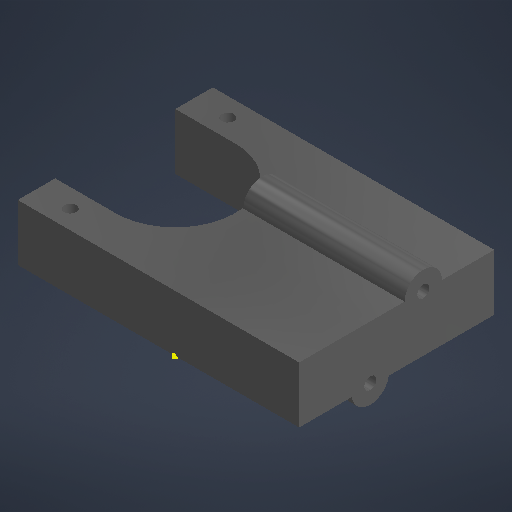
# Autodesk Inventor part: braket motor1
Saved by Autodesk Inventor 2026.2 (Build 302298010, 298A)
## iProperties
Part Number: braket motor1
Material: Generic
Document SubType Name: Modeling
Designer: acer
Appearance: Default
Author: acer
Autodesk Inventor part; units mm, degrees
ref_plane "YZ Plane" through (0, 0, 0) normal (1, 0, 0) x (0, 1, 0)
ref_plane "XZ Plane" through (0, 0, 0) normal (0, 1, 0) x (-1, 0, 0)
ref_plane "XY Plane" through (0, 0, 0) normal (0, 0, 1) x (1, 0, 0)
sketch "Sketch4" plane through (0, 0, 0) normal (0, 1, 0) x (-1, 0, 0)
  line L0 (0, 0) -> (-42, 0)
  line L1 (-42, 0) -> (-42, -52)
  line L2 (-42, -52) -> (0, -52)
  line L3 (0, -52) -> (0, 0)
  dimension "d79" = 42
  dimension "d80" = 52
  constraints: 8 end point, 2 parallel, 1 horizontal, 1 perpendicular
  measures "d79" distance of L2.end L1.end
  measures "d80" distance of L1.end L0.end
extrude "Extrusion4" add sketch "Sketch4" along normal blind 15
sketch "Sketch5" plane through (0, 15, 0) normal (0, 1, 0) x (1, 0, 0)
  line L0 (0, 0) -> (0, 10)
  line L1 (0, 52) -> (0, 0) projected
  line L2 (0, 52) -> (0, 42)
  circle A0 centre (16, 26) radius 16
  line L3 (42, 0) -> (42, 52) projected
  line L4 (0, 10) -> (42, 10)
  line L5 (0, 42) -> (42, 42)
  point P0 (42, 26)
  point P1 (16, 10)
  point P2 (16, 42)
  dimension "d83" = 10
  dimension "d84" = 10
  dimension "d93" = 32
  dimension "d94" = 26
  constraints: 8 end point, 4 point on line, 2 perpendicular, 1 centre point, 1 midpoint
  measures "d83" distance of L0.start L0.end
  measures "d84" distance of L1.start L2.end
  measures "d93" diameter of A0
  measures "d94" distance of point (42, 26) A0.centre
extrude "Extrusion5" cut sketch "Sketch5" against normal blind 15 contours L5 A0 L1 | A0 L4 L1 | A0
sketch "Sketch10" plane through (42, 0, 0) normal (1, 0, 0) x (0, 0, -1)
  circle A0 centre (5, 7.5) radius 2.65 projected
  line L0 (18.9423, 0.7517) -> (33.0845, 14.8938)
  line L1 (0, 0) -> (52, 0) projected
  line L2 (26, 0) -> (26, 15)
  line L3 (0, 15) -> (52, 15) projected
  line L4 (18.9423, 0.7517) -> (26.0134, 7.8228)
  circle A1 centre (18.9423, 0.7517) radius 1.55
  circle A2 centre (33.0845, 14.8938) radius 1.55
  circle A3 centre (33.0845, 14.8938) radius 5
  circle A4 centre (18.9423, 0.7517) radius 5
  line L5 (52, 0) -> (0, 0)
  point P0 (38.0833, 15)
  point P1 (28.0856, 15)
  point P2 (31.5381, 15)
  point P3 (34.6308, 15)
  point P4 (13.9992, 0)
  point P5 (23.8855, 0)
  point P6 (20.2979, 0)
  point P7 (17.5868, 0)
  point P8 (47, 7.5)
  dimension "d115" = 20
  dimension "d116" = 3.1
  dimension "d117" = 3.1
  dimension "d118" = 10
  dimension "d119" = 10
  constraints: 8 end point, 4 centre point, 4 coincident, 3 midpoint, 3 symmetric about line
  measures "d115" distance of L0.start L0.end
  measures "d116" diameter of A1
  measures "d117" diameter of A2
  measures "d118" diameter of A3
  measures "d119" diameter of A4
extrude "Extrusion10" add sketch "Sketch10" against normal blind 10 contours A1 L1 A4 | A3 L3 A2
sketch "Sketch11" plane through (42, 0, 0) normal (1, 0, 0) x (0, 0, -1)
  arc A0 (34.6308, 15) -> (31.5381, 15) centre (33.0845, 14.8938) ccw projected
  circle A1 centre (33.0845, 14.8938) radius 1.55
  point P0 (0, 0)
  point P1 (31.5381, 15)
  point P2 (34.6308, 15)
  dimension "d122" = 3.1
  constraints: 1 centre point, 1 coincident
  measures "d122" diameter of A1
extrude "Extrusion11" cut sketch "Sketch11" against normal blind 30
sketch "Sketch12" plane through (42, 0, 0) normal (1, 0, 0) x (0, 0, -1)
  circle A0 centre (33.0845, 14.8938) radius 1.55 projected
  circle A1 centre (33.0845, 14.8938) radius 3
  point P0 (0, 0)
  dimension "d125" = 6
  constraints: 1 centre point, 1 coincident
  measures "d125" diameter of A1
extrude "Extrusion12" cut sketch "Sketch12" against normal blind 30
sketch "Sketch13" plane through (42, 0, 0) normal (1, 0, 0) x (0, 0, -1)
  circle A0 centre (33.0845, 14.8938) radius 3 projected
  circle A1 centre (33.0845, 14.8938) radius 1.625
  point P0 (0, 0)
  dimension "d128" = 3.25
  constraints: 1 centre point, 1 coincident
  measures "d128" diameter of A1
extrude "Extrusion13" add sketch "Sketch13" against normal blind 5
sketch "Sketch14" plane through (42, 0, 0) normal (1, 0, 0) x (0, 0, -1)
  arc A0 (17.5868, 0) -> (20.2979, 0) centre (18.9423, 0.7517) ccw projected
  circle A1 centre (18.9423, 0.7517) radius 3
  point P0 (0, 0)
  dimension "d131" = 6
  constraints: 1 centre point, 1 coincident
  measures "d131" diameter of A1
extrude "Extrusion14" cut sketch "Sketch14" against normal blind 16
sketch "Sketch15" plane through (42, 0, 0) normal (1, 0, 0) x (0, 0, -1)
  circle A0 centre (18.9423, 0.7517) radius 1.625
  circle A1 centre (18.9423, 0.7517) radius 2.65
  point P0 (0, 0)
  dimension "d134" = 3.25
  constraints: 2 centre point, 2 coincident
  measures "d134" diameter of A0
extrude "Extrusion15" add sketch "Sketch15" against normal blind 5
sketch "Sketch16" plane through (42, 0, -52) normal (1, 0, 0) x (0, 0, -1)
  arc A0 (-20.2979, 0) -> (-17.5868, 0) centre (-18.9423, 0.7517) ccw projected
  circle A1 centre (-18.9423, 0.7517) radius 1.55
  point P0 (-52, 0)
  constraints: 1 centre point, 1 coincident
sketch "Sketch18" plane through (0, 0, 0) normal (0, -1, 0) x (1, 0, 0)
  line L0 (0, -10) -> (0, 0) projected
  line L1 (0, -5) -> (9, -5)
  circle A0 centre (9, -5) radius 1.625
  line L2 (0, -52) -> (0, -42) projected
  line L3 (0, -47) -> (9, -47)
  circle A1 centre (9, -47) radius 1.625
  dimension "d144" = 9
  dimension "d145" = 3.25
  dimension "d146" = 9
  dimension "d147" = 3.25
  constraints: 4 end point, 2 centre point, 2 coincident, 2 horizontal, 2 midpoint
  measures "d144" distance of L1.start L1.end
  measures "d145" diameter of A0
  measures "d146" distance of L3.start L3.end
  measures "d147" diameter of A1
extrude "Extrusion17" cut sketch "Sketch18" against normal blind 26.5
sketch "Sketch19" plane through (42, 0, 0) normal (1, 0, 0) x (0, 0, -1)
  point P0 (0, 0)
sketch "Sketch20" plane through (42, 0, 0) normal (1, 0, 0) x (0, 0, -1)
  point P0 (0, 0)
sketch "Sketch21" plane through (42, 0, 0) normal (1, 0, 0) x (0, 0, -1)
  line L0 (52, 0) -> (42, 0) projected
  line L1 (10, 15) -> (0, 15) projected
  line L2 (52, 0) -> (0, 0)
  line L3 (0, 0) -> (0, 15)
  line L4 (0, 15) -> (52, 15)
  line L5 (52, 15) -> (52, 0)
  circle A0 centre (18.9423, 0.7517) radius 1.625 projected
  circle A1 centre (18.9423, 0.7517) radius 1.625
  circle A2 centre (33.0845, 14.8938) radius 1.625
  circle A3 centre (33.0845, 14.8938) radius 1.625
  arc A4 (38.0833, 15) -> (28.0856, 15) centre (33.0845, 14.8938) ccw projected
  circle A5 centre (33.0845, 14.8938) radius 5
  arc A6 (13.9992, 0) -> (23.8855, 0) centre (18.9423, 0.7517) ccw projected
  circle A7 centre (18.9423, 0.7517) radius 5
  dimension "d150" = 3.25
  constraints: 8 end point, 5 coincident, 4 centre point, 2 parallel, 1 concentric, 1 horizontal, 1 perpendicular, 3 other
  measures "d150" diameter of A2
extrude "Extrusion18" add sketch "Sketch21" along normal blind 33 contours L0 L2 A7 L3 L1 L4 A5 L5 | A6 L2 A0 | L2 A0 A7 | A5 L4 A2 | L4 A2 A4
sketch "Sketch22" plane through (37, 0.7517, -18.9423) normal (-1, 0, 0) x (0, 0, 1)
  circle A0 centre (0, 0) radius 3 projected
  circle A1 centre (0, 0) radius 3
  point P0 (18.9423, -0.7517)
  dimension "d153" = 6
  constraints: 1 centre point, 1 coincident
  measures "d153" diameter of A1
extrude "Extrusion19" cut sketch "Sketch22" against normal blind 33
sketch "Sketch23" plane through (37, 14.8938, -33.0845) normal (-1, 0, 0) x (0, 0, 1)
  arc A0 (4.9989, 0.1062) -> (-4.9989, 0.1062) centre (0, 0) ccw projected
  circle A1 centre (0, 0) radius 3
  point P0 (33.0845, -14.8938)
  dimension "d156" = 6
  constraints: 1 centre point, 1 coincident
  measures "d156" diameter of A1
extrude "Extrusion20" cut sketch "Sketch23" against normal blind 33
body "Solid2"
